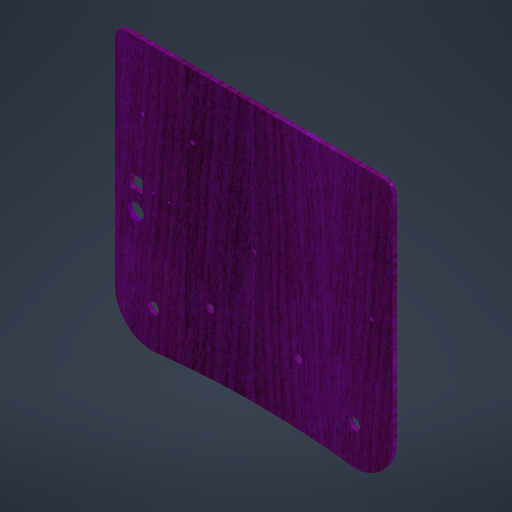
# Autodesk Inventor part: FTC Outside Panels
Saved by Autodesk Inventor 2024.2 (Build 282272000, 272)
## iProperties
Created: 2022-09-22
Part Number: FTC Outside Panels
Material: Wood (Oak)
Document SubType Name: Modeling
Designer: Jason
Density: 0.76 g/cm^3
Appearance: White Oak - Natural Medium Gloss
Author: Jason
Autodesk Inventor part; units mm, degrees
ref_plane "YZ Plane" through (0, 0, 0) normal (1, 0, 0) x (0, 1, 0)
ref_plane "XZ Plane" through (0, 0, 0) normal (0, 1, 0) x (-1, 0, 0)
ref_plane "XY Plane" through (0, 0, 0) normal (0, 0, 1) x (1, 0, 0)
sketch "Sketch1" plane through (0, 0, 0) normal (0, 0, 1) x (1, 0, 0)
  line L0 (0, 0) -> (333.375, 0)
  line L1 (333.375, 0) -> (333.375, 304.8)
  line L2 (320.675, 317.5) -> (12.7, 317.5)
  line L3 (0, 304.8) -> (0, 0)
  circle A0 centre (45.72, 45.72) radius 45.72
  circle A1 centre (287.655, 45.72) radius 45.72
  line L4 (166.6875, 0) -> (166.6875, 7.62)
  arc A2 (287.655, 0) -> (45.72, 0) centre (166.6875, -956.3695) ccw
  arc A3 (12.7, 317.5) -> (0, 304.8) centre (12.7, 304.8) ccw
  arc A4 (333.375, 304.8) -> (320.675, 317.5) centre (320.675, 304.8) ccw
  circle A5 centre (45.72, 45.72) radius 2.413
  circle A6 centre (287.655, 45.72) radius 2.413
  circle A7 centre (307.975, 165.1) radius 2.413
  line L5 (25.4, 165.1) -> (307.975, 165.1)
  circle A8 centre (166.6875, 165.1) radius 2.413
  line L6 (45.72, 45.72) -> (113.792, 45.72)
  line L7 (287.655, 45.72) -> (219.583, 45.72)
  line L8 (49.3862, 39.37) -> (53.0523, 45.72)
  line L9 (49.3862, 52.07) -> (53.0523, 45.72)
  line L10 (42.0538, 39.37) -> (49.3862, 39.37)
  line L11 (42.0538, 52.07) -> (49.3862, 52.07)
  line L12 (42.0538, 52.07) -> (38.3877, 45.72)
  line L13 (38.3877, 45.72) -> (42.0538, 39.37)
  line L14 (291.1818, 39.37) -> (294.848, 45.72)
  line L15 (291.1818, 52.07) -> (294.848, 45.72)
  line L16 (283.8495, 39.37) -> (291.1818, 39.37)
  line L17 (283.8495, 52.07) -> (291.1818, 52.07)
  line L18 (283.8495, 52.07) -> (280.1833, 45.72)
  line L19 (280.1833, 45.72) -> (283.8495, 39.37)
  line L20 (42.0538, 52.07) -> (49.3862, 39.37)
  line L21 (42.0538, 39.37) -> (49.3862, 52.07)
  line L22 (113.792, 95.337) -> (113.792, 63.3371)
  line L23 (113.792, 45.72) -> (113.792, 63.3371)
  circle A9 centre (113.792, 79.3371) radius 4.699
  ellipse E0 centre (113.792, 63.3371) end of major axis (113.7846, 65.3371) minor radius 2
  line L24 (219.583, 45.72) -> (219.583, 63.3371)
  ellipse E1 centre (219.583, 63.3371) end of major axis (219.5756, 65.3371) minor radius 2
  line L25 (219.583, 95.3392) -> (219.583, 63.3371)
  circle A10 centre (219.583, 79.3382) radius 4.699
  ellipse E2 centre (235.5574, 128.7087) end of major axis (235.56, 127.3562) minor radius 1.3525
  ellipse E3 centre (203.5575, 128.6472) end of major axis (203.5601, 127.2947) minor radius 1.3525
  ellipse E4 centre (219.583, 95.337) end of major axis (219.5791, 97.337) minor radius 2
  ellipse E5 centre (129.4616, 128.6451) end of major axis (129.4642, 127.2925) minor radius 1.3525
  ellipse E6 centre (97.4617, 128.6451) end of major axis (97.4643, 127.2925) minor radius 1.3525
  ellipse E7 centre (113.792, 95.337) end of major axis (113.7881, 97.337) minor radius 2
  line L26 (25.4, 165.1) -> (25.4, 157.48)
  line L27 (25.4, 157.48) -> (17.78, 157.48)
  line L28 (17.78, 157.48) -> (17.78, 165.1)
  line L29 (17.78, 165.1) -> (17.78, 172.72)
  line L30 (17.78, 172.72) -> (33.02, 172.72)
  line L31 (33.02, 172.72) -> (33.02, 157.48)
  line L32 (33.02, 157.48) -> (25.4, 157.48)
  point P0 (333.375, 317.5)
  point P1 (0, 317.5)
  point P2 (0, 0)
  point P3 (333.375, 45.72)
  point P4 (0, 45.72)
  point P5 (45.3639, 35.0229)
  point P6 (45.3639, 35.0229)
  point P7 (287.655, 45.72)
  point P8 (287.655, 45.72)
  point P9 (49.2468, 52.07)
  point P10 (291.1818, 52.07)
  point P11 (49.7423, 75.4671)
  point P12 (291.1818, 64.77)
  point P13 (45.72, 45.72)
  dimension "d176" = 91.44
  dimension "d177" = 91.44
  dimension "d174" = 333.375
  dimension "d175" = 317.5
  dimension "d178" = 7.62
  dimension "d179" = 12.7
  dimension "d180" = 4.826
  dimension "d181" = 4.826
  dimension "d184" = 25.4
  dimension "d185" = 4.826
  dimension "d186" = 25.4
  dimension "d188" = 4.826
  dimension "d193" = 68.072
  dimension "d194" = 68.072
  dimension "d195" = 165.1
  dimension "d206" = 12.7
  dimension "d207" = 12.7
  dimension "d208" = 12.7
  dimension "d209" = 7.3323
  dimension "d210" = 7.3323
  dimension "d211" = 7.3323
  dimension "d212" = 7.3323
  dimension "d213" = 7.3323
  dimension "d214" = 7.3323
  dimension "d215" = 12.7
  dimension "d216" = 12.7
  dimension "d217" = 12.7
  dimension "d218" = 7.3323
  dimension "d219" = 7.3323
  dimension "d220" = 7.3323
  dimension "d221" = 7.3323
  dimension "d222" = 7.3323
  dimension "d223" = 7.3323
  dimension "d224" = 17.6171
  dimension "d225" = 17.6171
  dimension "d226" = 9.398
  dimension "d227" = 9.398
  dimension "d228" = 31.9999
  dimension "d229" = 33.308
  dimension "d230" = 31.9999
  dimension "d231" = 33.308
  dimension "d232" = 15.6696
  dimension "d233" = 16.0255
  dimension "d234" = 31.9999
  dimension "d235" = 31.9999
  dimension "d236" = 180
  dimension "d237" = 0
  dimension "d258" = 7.62
  dimension "d259" = 7.62
  dimension "d260" = 7.62
  dimension "d261" = 7.62
  dimension "d262" = 15.24
  constraints: 66 end point, 13 centre point, 9 horizontal, 8 point on line, 7 point on circle, 7 vertical, 6 coincident, 6 perpendicular, 5 midpoint, 4 tangent, 2 parallel, 1 equal radius, 14 other
  measures "d174" distance of point (0, 317.5) point (333.375, 317.5)
  measures "d175" distance of point (333.375, 317.5) L0.end
  measures "d178" distance of L4.start L4.end
  measures "d179" radius of A3
  measures "d180" diameter of A5
  measures "d181" diameter of A6
  measures "d184" distance from line of L3 L5.start
  measures "d185" diameter of A7
  measures "d186" distance from line of L1 L5.end
  measures "d188" diameter of A8
  measures "d193" distance of L6.start L6.end
  measures "d194" distance of L7.start L7.end
  measures "d195" distance between parallel lines of L0 L5
  measures "d206" distance between parallel lines of L9 L13
  measures "d207" distance between parallel lines of L12 L8
  measures "d208" distance between parallel lines of L11 L10
  measures "d209" distance of L12.start L13.start
  measures "d210" distance of L13.start L10.start
  measures "d211" distance of L8.start L8.end
  measures "d212" distance of L10.start L8.start
  measures "d213" distance of L9.start L8.end
  measures "d214" distance of L12.start L11.end
  measures "d215" distance between parallel lines of L15 L19
  measures "d216" distance between parallel lines of L18 L14
  measures "d217" distance between parallel lines of L17 L16
  measures "d218" distance of L18.start L18.end
  measures "d219" distance of L18.end L19.end
  measures "d220" distance of L16.end L15.end
  measures "d221" distance of L19.end L16.end
  measures "d222" distance of L15.start L15.end
  measures "d223" distance of L18.start L17.end
  measures "d224" distance of L7.end L25.end
  measures "d225" distance of L6.end L22.end
  measures "d226" diameter of A10
  measures "d227" diameter of A9
  measures "d228" distance of E5.centre E6.centre
  measures "d229" vertical distance of L22.start E5.centre
  measures "d230" distance of E2.centre E3.centre
  measures "d231" vertical distance of L25.start E3.centre
  measures "d232" horizontal distance of E5.centre L22.start
  measures "d233" horizontal distance of point (219.583, 95.337) E3.centre
  measures "d234" distance of point (113.792, 63.337) L22.start
  measures "d235" distance of L25.end point (219.583, 95.337)
  measures "d236" angle of L25 L24
  measures "d237" vertical distance of E6.centre E5.centre
  measures "d258" distance of L5.start L26.end
  measures "d259" distance of L26.end L27.end
  measures "d260" distance of L27.end L28.end
  measures "d261" distance of L28.end L29.end
  measures "d262" distance of L29.end L30.end
extrude "Extrusion1" add sketch "Sketch1" along normal blind 5.08 contours A0 A2 | L3 A3 L2 A4 L1 A1 A2 A0 | A2 A1 | E0 L23 L22 | L22 L23 E0 | E1 L25 L24 | L24 L25 E1 | E2 | E3 | E4 | E5 | E6 | E7 picked at (16.5244, 31.421) picked at (316.8042, 60.019)
sketch "Sketch8" plane through (0, 0, 5.08) normal (0, 0, 1) x (1, 0, 0)
  line L0 (33.02, 172.72) -> (33.02, 157.48) projected
  line L1 (33.02, 157.48) -> (33.02, 165.1)
  line L2 (33.02, 165.1) -> (45.72, 165.1)
  line L3 (45.72, 165.1) -> (64.77, 165.1)
  circle A0 centre (64.9, 165.1) radius 1.3589
  circle A1 centre (45.85, 165.1) radius 1.3589
  line L4 (33.02, 165.1) -> (25.273, 165.1)
  line L5 (17.78, 157.48) -> (17.78, 172.72) projected
  point P0 (0, 0)
  dimension "d263" = 12.7
  dimension "d264" = 19.05
  dimension "d267" = 2.7178
  dimension "d268" = 2.7178
  dimension "d271" = 7.747
  constraints: 8 end point, 2 centre point, 2 perpendicular, 1 horizontal, 1 midpoint
  measures "d263" distance of L1.end L2.end
  measures "d264" distance of L2.end L3.end
  measures "d267" diameter of A0
  measures "d268" diameter of A1
  measures "d271" distance of L1.end L4.end
extrude "Extrusion8" cut sketch "Sketch8" against normal blind 28.5115
sketch "Sketch7" plane through (0, 0, 5.08) normal (0, 0, 1) x (1, 0, 0)
  line L0 (0, 304.8) -> (0, 45.72) projected
  line L1 (320.675, 317.5) -> (12.7, 317.5) projected
  circle A0 centre (33.02, 241.3) radius 2.413
  circle A1 centre (93.0148, 241.3) radius 2.413
  point P0 (0, 0)
  dimension "d243" = 4.826
  dimension "d244" = 4.826
  dimension "d245" = 76.2
  dimension "d246" = 33.02
  dimension "d247" = 59.9948
  dimension "d248" = 76.2
  constraints: 2 centre point
  measures "d243" diameter of A0
  measures "d244" diameter of A1
  measures "d245" distance from line of L1 A0.centre
  measures "d246" distance from line of L0 A0.centre
  measures "d247" distance of A1.centre A0.centre
  measures "d248" distance from line of L1 A1.centre
extrude "Extrusion10" cut sketch "Sketch7" against normal through all
sketch "Sketch9" plane through (0, 0, 5.08) normal (0, 0, 1) x (1, 0, 0)
  circle A0 centre (24.765, 135.255) radius 9.525
  line L0 (33.02, 157.48) -> (17.78, 157.48) projected
  line L1 (0, 304.8) -> (0, 45.72) projected
  point P0 (0, 0)
  dimension "d276" = 19.05
  dimension "d277" = 12.7
  dimension "d278" = 15.24
  constraints: 1 centre point
  measures "d276" diameter of A0
  measures "d277" distance edge to line of A0 L0
  measures "d278" distance edge to line of A0 L1
extrude "Extrusion11" cut sketch "Sketch9" against normal through all
body "Solid1"
